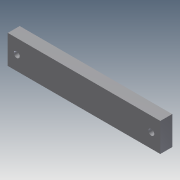
# Autodesk Inventor part: spacers
Saved by Autodesk Inventor 2011 (Build 150239000, 239)
## iProperties
Created: 2011-12-28
Part Number: spacers
Document SubType Name: Modeling
Designer: Matthew
Density: 1 g/cm^3
Author: Matthew
Autodesk Inventor part; units mm, degrees
ref_plane "YZ Plane" through (0, 0, 0) normal (1, 0, 0) x (0, 1, 0)
ref_plane "XZ Plane" through (0, 0, 0) normal (0, 1, 0) x (-1, 0, 0)
ref_plane "XY Plane" through (0, 0, 0) normal (0, 0, 1) x (1, 0, 0)
sketch "Sketch1" plane through (0, 0, 0) normal (0, 0, 1) x (1, 0, 0)
  line L0 (-36.9381, 4.4529) -> (64.6619, 4.4529)
  line L1 (64.6619, 4.4529) -> (64.6619, -14.5971)
  line L2 (64.6619, -14.5971) -> (-36.9381, -14.5971)
  line L3 (-36.9381, -14.5971) -> (-36.9381, 4.4529)
  point P0 (0, 0)
  dimension "d0" = 101.6
  dimension "d1" = 19.05
  constraints: 8 end point, 2 parallel, 1 horizontal, 1 perpendicular
  measures "d0" distance of L1.end L2.end
  measures "d1" distance of L0.end L1.end
extrude "Extrusion1" add sketch "Sketch1" along normal blind 7.9375
sketch "Sketch2" plane through (0, 0, 7.9375) normal (0, 0, 1) x (1, 0, 0)
  line L0 (-36.9381, -14.5971) -> (-36.9381, 4.4529) projected
  line L1 (64.6619, -14.5971) -> (-36.9381, -14.5971) projected
  line L2 (-36.9381, -5.0721) -> (13.8619, -5.0721)
  line L3 (13.8619, -5.0721) -> (58.6929, -5.0721)
  line L4 (58.6929, -5.0721) -> (-30.9691, -5.0721)
  circle A0 centre (-30.9691, -5.0721) radius 1.9812
  circle A1 centre (58.6929, -5.0721) radius 1.9812
  point P0 (0, 0)
  dimension "d4" = 44.831
  dimension "d5" = 89.662
  dimension "d6" = 3.9624
  constraints: 6 end point, 2 centre point, 2 coincident, 2 point on line, 1 midpoint, 1 parallel
  measures "d4" distance of L2.end L3.end
  measures "d5" distance of L3.end L4.end
  measures "d6" diameter of A0
extrude "Extrusion2" cut sketch "Sketch2" against normal blind 7.9375
body "Solid1"
